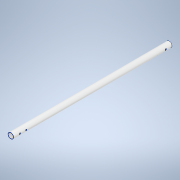
# Autodesk Inventor part: BodyTube
Saved by Autodesk Inventor 2022.1 (Build 261234020, 234B)
## iProperties
Created: 2021-11-14
Part Number: BodyTube
Material: Aluminum 6061
Document SubType Name: Modeling
Designer: Alexander
Density: 2.7 g/cm^3
Appearance: Aluminum - Flat
Mass: 71.8389 g
Surface Area: 534.065 cm^2
Volume: 26.607 cm^3
Author: Alexander
Autodesk Inventor part; units mm, degrees
ref_plane "YZ Plane" through (0, 0, 0) normal (1, 0, 0) x (0, 1, 0)
ref_plane "XZ Plane" through (0, 0, 0) normal (0, 1, 0) x (-1, 0, 0)
sketch "Sketch1" plane through (0, 0, 0) normal (0, 0, 1) x (1, 0, 0)
  circle A0 centre (0, 0) radius 8
  circle A1 centre (0, 0) radius 9
  dimension "d0" = 16
  dimension "d1" = 18
  constraints: 2 centre point, 2 coincident
  measures "d0" diameter of A0
  measures "d1" diameter of A1
extrude "Extrusion1" add sketch "Sketch1" along normal blind 500
ref_plane "Work Plane2" through (5.5, 0, -32) normal (1, 0, 0) x (0, 0, 1)
sketch "Sketch2" plane through (5.5, 0, -32) normal (1, 0, 0) x (0, 0, 1)
  circle A0 centre (52, 0) radius 2.25
  line L0 (32, -9) -> (32, 9) projected
  circle A1 centre (512, 0) radius 2.25
  circle A2 centre (492, 0) radius 2.25
  line L1 (532, -9) -> (532, 9) projected
  point P0 (32, 0)
  dimension "d4" = 4.5
  dimension "d5" = 20
  dimension "d8" = 4.5
  dimension "d9" = 4.5
  dimension "d10" = 20
  dimension "d11" = 20
  constraints: 3 centre point
  measures "d4" diameter of A0
  measures "d5" distance from line of L0 A0.centre
  measures "d8" diameter of A1
  measures "d9" diameter of A2
  measures "d10" distance from line of L1 A1.centre
  measures "d11" distance of A1.centre A2.centre
extrude "Extrusion2" cut sketch "Sketch2" along normal through all both and the other way through all
body "Solid1"
